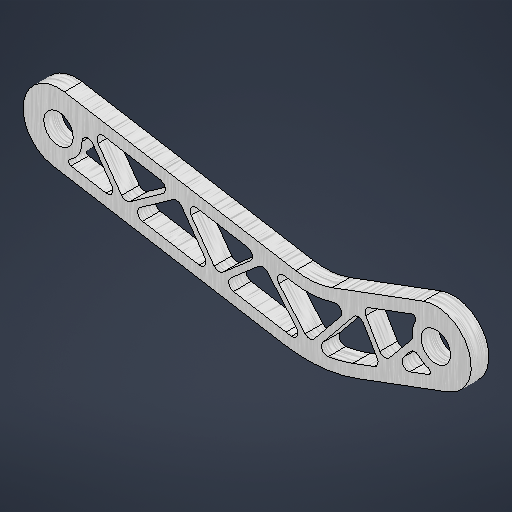
# Autodesk Inventor part: PLATE,LINK,FRONT,INTAKE
Saved by Autodesk Inventor 2026 (Build 300175000, 175)
## iProperties
Created: 2026-02-15
Part Number: PLATE,LINK,FRONT,INTAKE
Material: Aluminum 7075
Document SubType Name: Modeling
Designer: Jthib
Mass: 133.983 g
Surface Area: 232.016 cm^2
Volume: 47.6809 cm^3
Density: 2.81 g/cm^3
Appearance: Satin - Brushed Heavy
Author: Jthib
Autodesk Inventor part; units mm, degrees
ref_plane "YZ Plane" through (0, 0, 0) normal (1, 0, 0) x (0, 1, 0)
ref_plane "XZ Plane" through (0, 0, 0) normal (0, 1, 0) x (-1, 0, 0)
sketch "Sketch1" plane through (0, 0, 0) normal (0, 0, 1) x (1, 0, 0)
  line L0 (-101.6, 0) -> (101.6, 0) construction
  arc A0 (-98.4242, 18.7834) -> (-104.7758, -18.7834) centre (-101.6, 0) ccw
  arc A1 (108.2414, -17.8548) -> (94.9586, 17.8548) centre (101.6, 0) ccw
  line L1 (108.2414, -17.8548) -> (59.0939, -36.136)
  line L2 (19.8252, -39.8504) -> (-104.7758, -18.7834)
  line L3 (-98.4242, 18.7834) -> (26.1768, -2.2835)
  line L4 (45.8112, -0.4263) -> (94.9586, 17.8548)
  line L5 (36.2428, -3.9854) -> (39.9572, -43.2542) construction
  line L6 (38.1, -23.6198) -> (-101.6, 0) construction
  line L7 (38.1, -23.6198) -> (101.6, 0) construction
  arc A2 (19.8252, -39.8504) -> (59.0939, -36.136) centre (32.5284, 35.2833) ccw
  arc A3 (26.1768, -2.2835) -> (45.8112, -0.4263) centre (32.5284, 35.2833) ccw
  point P0 (0, 0)
  dimension "d1" = 38.1
  dimension "d2" = 203.2
  dimension "d12" = 150
  dimension "d13" = 63.5
  dimension "d14" = 76.2
  constraints: 18 end point, 8 point on circle, 8 tangent, 4 centre point, 4 point on line, 2 midpoint, 2 parallel, 1 concentric, 1 equal radius, 1 horizontal
  measures "d1" diameter of A0
  measures "d2" distance of L0.start L0.end
  measures "d12" angle of L7 L6
  measures "d13" horizontal distance of L6.start L0.end
  measures "d14" radius of A2
extrude "Extrusion1" add sketch "Sketch1" along normal mid plane 9.525
sketch "Sketch2" plane through (0, 0, 4.7625) normal (0, 0, 1) x (1, 0, 0)
  arc A0 (-98.4242, 18.7834) -> (-104.7758, -18.7834) centre (-101.6, 0) ccw construction
  arc A1 (108.2414, -17.8548) -> (94.9586, 17.8548) centre (101.6, 0) ccw construction
  point P0 (0, 0)
  constraints: 2 coincident
hole "Hole1" at (-101.6, 0, 4.7625) at (101.6, 0, 4.7625) direction (0, 0, -1) diameter 15.875 end through all
sketch "Sketch3" plane through (0, 0, -4.7625) normal (0, 0, -1) x (-1, 0, 0)
  circle A0 centre (-101.6, 0) radius 7.9375 projected
  circle A1 centre (101.6, 0) radius 7.9375 projected
  line L0 (-19.8252, -39.8504) -> (104.7758, -18.7834) projected
  arc A2 (104.7758, -18.7834) -> (98.4242, 18.7834) centre (101.6, 0) ccw projected
  line L1 (98.4242, 18.7834) -> (-26.1768, -2.2835) projected
  arc A3 (-45.8112, -0.4263) -> (-26.1768, -2.2835) centre (-32.5284, 35.2833) ccw projected
  line L2 (-45.8112, -0.4263) -> (-94.9586, 17.8548) projected
  arc A4 (-94.9586, 17.8548) -> (-108.2414, -17.8548) centre (-101.6, 0) ccw projected
  line L3 (-108.2414, -17.8548) -> (-59.0939, -36.136) projected
  arc A5 (-59.0939, -36.136) -> (-19.8252, -39.8504) centre (-32.5284, 35.2833) ccw projected
  line L4 (103.7172, -12.5223) -> (-20.8838, -33.5892)
  arc A6 (-56.8801, -30.1844) -> (-20.8838, -33.5892) centre (-32.5284, 35.2833) ccw
  line L5 (-56.8801, -30.1844) -> (-106.0276, -11.9032)
  arc A7 (-97.1724, 11.9032) -> (-106.0276, -11.9032) centre (-101.6, 0) ccw
  line L6 (-97.1724, 11.9032) -> (-48.025, -6.3779)
  arc A8 (-48.025, -6.3779) -> (-25.1182, -8.5447) centre (-32.5284, 35.2833) ccw
  line L7 (-25.1182, -8.5447) -> (99.4828, 12.5223)
  arc A9 (103.7172, -12.5223) -> (99.4828, 12.5223) centre (101.6, 0) ccw
  circle A10 centre (101.6, 0) radius 12.7
  circle A11 centre (-101.6, 0) radius 12.7
  point P0 (0, 0)
  point P1 (-97.1724, 11.9032)
  dimension "d16" = 6.35
  constraints: 8 end point, 8 point on circle, 6 centre point, 2 concentric, 7 other
  measures "d16" distance between parallel lines of L0 L4
extrude "Extrusion2" cut sketch "Sketch3" against normal through all contours L4 A6 L5 A11 L6 A8 L7 A10
sketch "Sketch4" plane through (0, 0, -4.7625) normal (0, 0, -1) x (-1, 0, 0)
  arc A0 (99.4828, 12.5223) -> (103.7172, -12.5223) centre (101.6, 0) ccw projected
  line L0 (103.7172, -12.5223) -> (-20.8838, -33.5892) projected
  arc A1 (-56.8801, -30.1844) -> (-20.8838, -33.5892) centre (-32.5284, 35.2833) ccw projected
  line L1 (-56.8801, -30.1844) -> (-106.0276, -11.9032) projected
  arc A2 (-106.0276, -11.9032) -> (-97.1724, 11.9032) centre (-101.6, 0) ccw projected
  line L2 (-97.1724, 11.9032) -> (-48.025, -6.3779) projected
  arc A3 (-48.025, -6.3779) -> (-25.1182, -8.5447) centre (-32.5284, 35.2833) ccw projected
  line L3 (-25.1182, -8.5447) -> (99.4828, 12.5223) projected
  circle A4 centre (-101.6, 0) radius 7.9375 projected
  circle A5 centre (101.6, 0) radius 7.9375 projected
  line L4 (-19.8252, -39.8504) -> (104.7758, -18.7834) projected
  arc A6 (104.7758, -18.7834) -> (98.4242, 18.7834) centre (101.6, 0) ccw projected
  line L5 (98.4242, 18.7834) -> (-26.1768, -2.2835) projected
  arc A7 (-45.8112, -0.4263) -> (-26.1768, -2.2835) centre (-32.5284, 35.2833) ccw projected
  line L6 (-45.8112, -0.4263) -> (-94.9586, 17.8548) projected
  arc A8 (-94.9586, 17.8548) -> (-108.2414, -17.8548) centre (-101.6, 0) ccw projected
  line L7 (-108.2414, -17.8548) -> (-59.0939, -36.136) projected
  arc A9 (-59.0939, -36.136) -> (-19.8252, -39.8504) centre (-32.5284, 35.2833) ccw projected
  line L8 (101.6, 0) -> (86.9605, 10.4051)
  line L9 (86.9605, 10.4051) -> (66.1504, -18.8739)
  line L10 (66.1504, -18.8739) -> (36.8714, 1.9362)
  line L11 (-25.1182, -8.5447) -> (99.4828, 12.5223) projected
  line L12 (36.8714, 1.9362) -> (16.0613, -27.3427)
  line L13 (-33.7195, -34.5565) -> (-60.4545, -1.7546)
  line L14 (-60.4545, -1.7546) -> (-73.5074, -23.9996)
  line L15 (-73.5074, -23.9996) -> (-89.6968, -4.4276)
  line L16 (16.0613, -27.3427) -> (-8.8807, -5.7993)
  line L17 (-8.8807, -5.7993) -> (-33.7195, -34.5565)
  point P0 (0, 0)
  dimension "d20" = 90
  dimension "d21" = 30
  dimension "d22" = 45
  dimension "d23" = 80
  dimension "d24" = 70
  constraints: 18 end point, 7 point on line, 3 perpendicular, 3 point on circle, 1 coincident
  measures "d20" angle of L17 L16
  measures "d21" angle of L1 L15
  measures "d22" angle of L3 L8
  measures "d23" angle of L13 L17
  measures "d24" angle of L15 L14
ref_plane "Work Plane1" through (-101.6, 0, -4.7625) normal (0.8150928, 0.5793304, 0) x (-0.5793304, 0.8150928, 0)
sketch "Sketch5" plane through (-101.6, 0, -4.7625) normal (0.8150928, 0.5793304, 0) x (-0.5793304, 0.8150928, 0)
  line L0 (1.5875, 0) -> (-1.5875, 0)
  line L1 (-1.5875, 0) -> (-1.5875, 9.525)
  line L2 (-1.5875, 9.525) -> (1.5875, 9.525)
  line L3 (1.5875, 9.525) -> (1.5875, 0)
  line L4 (1.5875, 0) -> (-1.5875, 9.525) construction
  line L5 (-1.5875, 0) -> (1.5875, 9.525) construction
  point P0 (-58.86, 4.7625)
  point P1 (0, 4.7625)
  point P2 (0, 0)
  point P3 (0, 0)
  dimension "d25" = 9.525
  dimension "d26" = 3.175
  constraints: 12 end point, 3 midpoint, 2 parallel, 1 coincident, 1 horizontal, 1 perpendicular
  measures "d25" distance of L0.end L1.end
  measures "d26" distance of L1.end L2.end
sweep "Sweep1" add profiles "Sketch5" path "Sketch4" path curves L8 L9 L10 L12 L16 L17 L13 L14 L15
delete faces "Delete Face1" heal yes whole lump no faces at (89.289, -4.0903, 1.5875) (-101.2934, -0.4313, -1.5875) (-100.4067, 2.7958, 1.5875) (-98.5673, 0.2079, -1.5875) (-98.5709, 12.3335, -1.5875) (-96.0466, 11.9413, -1.5875) (-90.1992, 10.0508, 1.5875)
fillet "Fillet1" radius 3.175 26 edges at (-68.364, -18.4996, 0) (-87.3348, 8.1914, 0) (-90.4098, 6.0058, 0) (-39.0851, 2.3105, 0) (-84.7469, 10.0308, 0) (-63.9367, -19.2482, 0) (-65.7761, -16.6603, 0) (-18.2749, -26.9685, 0) (-37.2457, -0.2774, 0) (-34.6578, 1.562, 0) (-15.7783, -25.0006, 0) (6.8497, -5.4559, 0) (8.717, -8.0384, 0) (-14.0302, -27.6861, 0) (31.6256, -34.5609, 0) (35.8226, -34.489, 0) (33.6842, -32.0871, 0) (57.5155, -2.8478, 0) (11.3372, -6.2146, 0) (71.9965, -24.5616, 0) (60.2416, -4.5285, 0) (61.9654, -1.1926, 0) (73.7292, -21.2408, 0) (76.4832, -22.8927, 0) (89.1648, -2.58, 0) (90.4263, -6.0364, 0)
fillet "Fillet1" radius 1.5875 3 edges at (-103.7172, -12.5223, 0) (97.1724, 11.9032, 0) (106.0276, -11.9032, 0)
equation "\"d25\" = d3"
equation "\"d3\" = 9.525"
body "Solid1"
